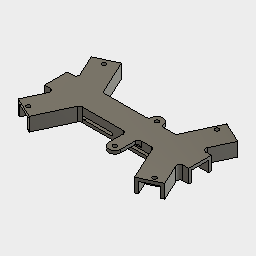
Central Frame V1.2 v4 (Autodesk Fusion 360 design; units mm, degrees)
Autodesk Fusion 360 part; units mm, degrees
sketch "Sketch1" plane through (0, 0, 0) normal (0, 1, 0) x (1, 0, 0)
  line L0 (13.8907, 50.6995) -> (18.8907, 50.6995) construction
  line L1 (13.8907, 50.6995) -> (21.3907, 50.6995) construction
  line L2 (20.688, 53.8691) -> (29.9066, 34.0997)
  line L3 (13.8907, 50.6995) -> (21.3907, 50.6995) construction
  line L4 (7.0934, 47.5298) -> (13.3559, 34.0997)
  line L5 (7.0934, 5.6696) -> (13.3559, 19.0997)
  line L6 (20.688, -0.6696) -> (29.9066, 19.0997)
  line L7 (7.0934, 47.5298) -> (4.9803, 52.0614)
  line L8 (7.0934, 47.5298) -> (12.0934, 47.5298) construction
  line L9 (4.9803, 52.0614) -> (18.5749, 58.4007)
  line L10 (20.688, 53.8691) -> (18.5749, 58.4007)
  line L11 (7.0934, 5.6696) -> (4.9803, 1.1381)
  line L12 (7.0934, 5.6696) -> (12.0934, 5.6696) construction
  line L13 (4.9803, 1.1381) -> (18.5749, -5.2012)
  line L14 (4.9803, 1.1381) -> (19.9803, 1.1381) construction
  line L15 (18.5749, -5.2012) -> (20.688, -0.6696)
  line L16 (13.3559, 34.0997) -> (13.3559, 19.0997)
  line L17 (96.6149, 2.5) -> (104.1149, 2.5) construction
  line L18 (85.1097, 49.1342) -> (78.099, 34.0997)
  line L19 (87.3176, -0.6696) -> (78.099, 19.0997)
  line L20 (94.6496, 34.0997) -> (94.6496, 19.0997)
  line L21 (100.9122, 5.6696) -> (94.6496, 19.0997)
  line L22 (100.9122, 47.5298) -> (94.6496, 34.0997)
  line L23 (103.0253, 52.0614) -> (89.4307, 58.4007)
  line L24 (100.9122, 47.5298) -> (103.0253, 52.0614)
  line L25 (87.3176, 53.8691) -> (89.4307, 58.4007)
  line L26 (100.9122, 5.6696) -> (103.0253, 1.1381)
  line L27 (103.0253, 1.1381) -> (89.4307, -5.2012)
  line L28 (89.4307, -5.2012) -> (87.3176, -0.6696)
  line L29 (29.9066, 34.0997) -> (60.3566, 34.0997)
  line L30 (68.3041, 34.0997) -> (78.099, 34.0997)
  arc A0 (68.3041, 35.3466) -> (60.3097, 35.3466) centre (64.3069, 35.4968) ccw
  line L31 (60.3097, 7.4466) -> (60.3097, 19.0997)
  line L32 (68.3069, 7.5968) -> (68.3069, 19.0997)
  arc A1 (60.3097, 7.747) -> (68.3069, 7.5968) centre (64.3069, 7.5968) ccw
  line L33 (29.9066, 19.0997) -> (60.3097, 19.0997)
  line L34 (68.3069, 19.0997) -> (78.099, 19.0997)
  line L35 (60.3097, 35.3466) -> (60.3566, 34.0997)
  line L36 (68.3041, 35.3466) -> (68.3041, 34.0989)
  line L37 (85.1097, 49.1342) -> (87.3176, 53.8691)
  dimension "d15" = 27.9
  dimension "d89" = 7.5
  dimension "d91" = 7.5
  dimension "d95" = 115
  dimension "d96" = 5
  dimension "d97" = 115
  dimension "d98" = 5
  dimension "d99" = 25
  dimension "d100" = 15
  dimension "d107" = 8
  dimension "d109" = 8
  dimension "d110" = 1.2478
  constraint horizontal L0
  constraint horizontal L1
  constraint horizontal L3
  constraint horizontal L8
  constraint perpendicular L2 L9
  constraint perpendicular L9 L10
  constraint horizontal L12
  constraint horizontal L14
  constraint perpendicular L13 L15
  constraint horizontal L29
  constraint horizontal L17
  constraint collinear L29 L30
  constraint coincident A1
  constraint perpendicular L31 L33
  constraint coincident origin L33
  constraint tangent L32 A1
  constraint perpendicular L32 L33
  constraint coincident L31
  constraint collinear L33 L34
  constraint tangent A0 L35
  constraint vertical L36
  constraint coincident L36
  constraint parallel L18 L37
  measures "d91" distance of origin
  measures "d95" angle of L7 L8
  measures "d97" angle of L11 L12
  measures "d98" distance of origin
  measures "d99" angle of L13 L14
  measures "d107" diameter of A0
  measures "d109" diameter of A1
  measures "d110" distance of origin
extrude "Extrude1" add sketch "Sketch1" along normal blind 2 contours L2 L4 L5 L6 L7 L9 L10 L11 L13 L15 L16 L18 L19 L20 L21 L22 L23 L24 L25 L26 L27 L28 L29 L30 A0 L31 L32 A1 L33 L34 L35 L36 L37
sketch "Sketch12" plane through (0, 2, 0) normal (0, 1, 0) x (-1, 0, 0)
  line L0 (-13.3559, -19.0997) -> (-4.9803, -1.1381)
  line L1 (-4.9803, -1.1381) -> (-18.5749, 5.2012)
  line L2 (-18.5749, 5.2012) -> (-29.9066, -19.0997)
  line L3 (-29.9066, -19.0997) -> (-60.3097, -19.0997)
  line L4 (-60.3097, -19.0997) -> (-60.3097, -7.4466)
  arc A0 (-60.3097, -7.4466) -> (-68.3069, -7.5968) centre (-64.3069, -7.5968) ccw
  line L5 (-68.3069, -7.5968) -> (-68.3069, -19.0997)
  line L6 (-68.3069, -19.0997) -> (-78.099, -19.0997)
  line L7 (-78.099, -19.0997) -> (-89.4307, 5.2012)
  line L8 (-89.4307, 5.2012) -> (-103.0253, -1.1381)
  line L9 (-103.0253, -1.1381) -> (-94.6496, -19.0997)
  line L10 (-94.6496, -19.0997) -> (-94.6496, -34.0997)
  line L11 (-94.6496, -34.0997) -> (-103.0253, -52.0614)
  line L12 (-103.0253, -52.0614) -> (-89.4307, -58.4007)
  line L13 (-89.4307, -58.4007) -> (-78.099, -34.0997)
  line L14 (-78.099, -34.0997) -> (-68.3041, -34.0997)
  line L15 (-68.3041, -34.0997) -> (-68.3041, -35.3466)
  arc A1 (-68.3041, -35.3466) -> (-60.3097, -35.3466) centre (-64.3069, -35.4968) ccw
  line L16 (-60.3097, -35.3466) -> (-60.3566, -34.0997)
  line L17 (-60.3566, -34.0997) -> (-29.9066, -34.0997)
  line L18 (-29.9066, -34.0997) -> (-18.5749, -58.4007)
  line L19 (-18.5749, -58.4007) -> (-4.9803, -52.0614)
  line L20 (-4.9803, -52.0614) -> (-13.3559, -34.0997)
  line L21 (-13.3559, -34.0997) -> (-13.3559, -19.0997)
  circle A2 centre (-13.0706, -1.5207) radius 1.3
  circle A3 centre (-13.8907, -50.6995) radius 1.3
  circle A4 centre (-64.3069, -7.5968) radius 1.3
  circle A5 centre (-64.3069, -35.4968) radius 1.3
  circle A6 centre (-88.7907, -50.6995) radius 1.3
  circle A7 centre (-95.7752, -2.3455) radius 1.3
  dimension "d193" = 2.6
  dimension "d194" = 2.6
  dimension "d195" = 2.6
  dimension "d196" = 2.6
  dimension "d197" = 2.6
  dimension "d198" = 2.6
  measures "d193" diameter of A2
  measures "d194" diameter of A3
  measures "d195" diameter of A4
  measures "d196" diameter of A5
  measures "d197" diameter of A6
  measures "d198" diameter of A7
extrude "Extrude10" cut sketch "Sketch12" against normal blind 2 contours A2 | A3 | A4 | A5 | A6 | A7
sketch "Sketch13" plane through (0, 0, 0) normal (0, -1, 0) x (1, 0, 0)
  line L0 (60.3566, -34.0997) -> (60.3097, -35.3466)
  arc A0 (60.3097, -35.3466) -> (68.3041, -35.3466) centre (64.3069, -35.4968) ccw
  line L1 (68.3041, -35.3466) -> (68.3041, -34.0997)
  line L2 (68.3041, -34.0997) -> (78.099, -34.0997)
  line L3 (78.099, -34.0997) -> (89.4307, -58.4007)
  line L4 (89.4307, -58.4007) -> (103.0253, -52.0614)
  line L5 (103.0253, -52.0614) -> (94.6496, -34.0997)
  line L6 (94.6496, -34.0997) -> (94.6496, -19.0997)
  line L7 (94.6496, -19.0997) -> (103.0253, -1.1381)
  line L8 (103.0253, -1.1381) -> (89.4307, 5.2012)
  line L9 (89.4307, 5.2012) -> (78.099, -19.0997)
  line L10 (78.099, -19.0997) -> (68.3069, -19.0997)
  line L11 (68.3069, -19.0997) -> (68.3069, -7.5968)
  arc A1 (68.3069, -7.5968) -> (60.3097, -7.4466) centre (64.3069, -7.5968) ccw
  line L12 (60.3097, -7.4466) -> (60.3097, -19.0997)
  line L13 (60.3097, -19.0997) -> (29.9066, -19.0997)
  line L14 (29.9066, -19.0997) -> (18.5749, 5.2012)
  line L15 (18.5749, 5.2012) -> (4.9803, -1.1381)
  line L16 (4.9803, -1.1381) -> (13.3559, -19.0997)
  line L17 (13.3559, -19.0997) -> (13.3559, -34.0997)
  line L18 (13.3559, -34.0997) -> (4.9803, -52.0614)
  line L19 (4.9803, -52.0614) -> (18.5749, -58.4007)
  line L20 (18.5749, -58.4007) -> (29.9066, -34.0997)
  line L21 (29.9066, -34.0997) -> (60.3566, -34.0997)
  line L22 (62.4331, -32.0997) -> (66.3041, -32.0997)
  line L23 (62.3097, -21.0997) -> (66.3069, -21.0997)
  line L24 (15.3559, -18.6563) -> (15.3559, -34.5431)
  line L25 (28.6325, -32.0997) -> (62.4331, -32.0997)
  line L26 (66.3041, -32.0997) -> (79.3731, -32.0997)
  line L27 (88.975, -52.691) -> (90.3981, -55.7428)
  line L28 (92.6496, -34.5431) -> (92.6496, -18.6563)
  line L29 (79.3731, -21.0997) -> (66.3069, -21.0997)
  line L30 (62.3097, -21.0997) -> (28.6325, -21.0997)
  line L31 (87.3836, -49.2782) -> (88.975, -52.691)
  line L32 (60.3566, -34.0997) -> (68.3041, -34.0997)
  line L33 (60.3097, -19.0997) -> (68.3069, -19.0997)
  line L34 (7.6381, -51.094) -> (6.7929, -52.9066)
  line L35 (17.6075, -55.7428) -> (16.7623, -57.5554)
  line L36 (17.6075, -55.7428) -> (19.6075, -55.7428) construction
  line L37 (7.6381, -2.1055) -> (6.7929, -0.2929)
  line L38 (17.6075, 2.5433) -> (16.7623, 4.3559)
  line L39 (17.6075, 2.5433) -> (19.6075, 2.5433) construction
  line L40 (90.3981, 2.5433) -> (91.2433, 4.3559)
  line L41 (90.3981, 2.5433) -> (92.3981, 2.5433) construction
  line L42 (100.3674, -2.1055) -> (101.2127, -0.2929)
  line L43 (100.3674, -2.1055) -> (102.3674, -2.1055) construction
  line L44 (90.3981, -55.7428) -> (91.2433, -57.5554)
  line L45 (90.3981, -55.7428) -> (92.3981, -55.7428) construction
  line L46 (100.3674, -51.094) -> (101.2127, -52.9066)
  line L47 (6.7929, -0.2929) -> (11.0191, -9.3559)
  line L48 (6.7929, -0.2929) -> (16.7929, -0.2929) construction
  line L49 (11.0191, -9.3559) -> (20.9885, -4.7071)
  line L50 (6.7929, -52.9066) -> (11.0191, -43.8435)
  line L51 (6.7929, -52.9066) -> (16.7929, -52.9066) construction
  line L52 (11.0191, -43.8435) -> (20.9885, -48.4923)
  line L53 (91.2433, 4.3559) -> (87.0171, -4.7071)
  line L54 (87.0171, -4.7071) -> (96.9865, -9.3559)
  line L55 (101.2127, -52.9066) -> (96.9865, -43.8435)
  line L56 (101.2127, -52.9066) -> (111.2127, -52.9066) construction
  line L57 (96.9865, -43.8435) -> (87.0171, -48.4923)
  line L58 (11.497, -42.8186) -> (21.4664, -47.4674)
  line L59 (11.497, -10.3809) -> (21.4664, -5.7321)
  line L60 (86.5392, -5.7321) -> (96.5085, -10.3809)
  line L61 (96.5085, -42.8186) -> (86.5392, -47.4674)
  line L62 (17.6075, -55.7428) -> (20.9885, -48.4923)
  line L63 (21.4664, -47.4674) -> (28.6325, -32.0997)
  line L64 (15.3559, -34.5431) -> (11.497, -42.8186)
  line L65 (11.0191, -43.8435) -> (7.6381, -51.094)
  line L66 (7.6381, -2.1055) -> (11.0191, -9.3559)
  line L67 (11.497, -10.3809) -> (15.3559, -18.6563)
  line L68 (28.6325, -21.0997) -> (21.4664, -5.7321)
  line L69 (20.9885, -4.7071) -> (17.6075, 2.5433)
  line L70 (90.3981, 2.5433) -> (87.0171, -4.7071)
  line L71 (86.5392, -5.7321) -> (79.3731, -21.0997)
  line L72 (92.6496, -18.6563) -> (96.5085, -10.3809)
  line L73 (96.9865, -9.3559) -> (100.3674, -2.1055)
  line L74 (100.3674, -51.094) -> (96.9865, -43.8435)
  line L75 (96.5085, -42.8186) -> (92.6496, -34.5431)
  line L76 (79.3731, -32.0997) -> (86.5392, -47.4674)
  line L77 (87.0171, -48.4923) -> (87.3836, -49.2782)
  circle A2 centre (88.7907, -50.6995) radius 1.3
  circle A3 centre (13.0706, -1.5207) radius 1.3
  circle A4 centre (64.3069, -35.4968) radius 1.3
  circle A5 centre (95.7752, -2.3455) radius 1.3
  circle A6 centre (64.3069, -7.5968) radius 1.3
  circle A7 centre (13.8907, -50.6995) radius 1.3
  dimension "d131" = 115
  dimension "d132" = 2
  dimension "d133" = 115
  dimension "d134" = 2
  dimension "d135" = 115
  dimension "d136" = 2
  dimension "d137" = 65
  dimension "d138" = 2
  dimension "d139" = 65
  dimension "d140" = 2
  dimension "d141" = 65
  dimension "d142" = 2
  dimension "d143" = 65
  dimension "d144" = 10
  dimension "d145" = 65
  dimension "d146" = 10
  dimension "d147" = 10
  dimension "d148" = 115
  dimension "d149" = 10
  constraint parallel L16 L66
  constraint parallel L17 L24
  constraint parallel L18 L64
  constraint parallel L20 L62
  constraint parallel L21 L25
  constraint parallel L2 L26
  constraint parallel L3 L27
  constraint parallel L5 L74
  constraint parallel L6 L28
  constraint parallel L7 L72
  constraint parallel L9 L70
  constraint parallel L10 L29
  constraint parallel L13 L30
  constraint parallel L14 L68
  constraint parallel L27 L31
  constraint coincident L19 origin
  constraint horizontal L36
  constraint horizontal L39
  constraint horizontal L41
  constraint horizontal L43
  constraint horizontal L45
  constraint coincident L4 origin
  constraint horizontal L48
  constraint coincident origin L68
  constraint perpendicular L49 L68
  constraint horizontal L51
  constraint perpendicular L52 L62
  constraint coincident L72
  constraint perpendicular L54 L72
  constraint horizontal L56
  constraint coincident origin L76
  constraint perpendicular L57 L76
  constraint coincident origin L62
  constraint perpendicular L58 L62
  constraint perpendicular L59 L66
  constraint coincident L70
  constraint perpendicular L60 L72
  constraint perpendicular L61 L76
  constraint collinear L62 L63
  constraint collinear L64 L65
  constraint collinear L66 L67
  constraint coincident L66
  constraint collinear L68 L69
  constraint collinear L70 L71
  constraint collinear L72 L73
  constraint collinear L74 L75
  constraint coincident L74
  constraint collinear L76 L77
  measures "d131" angle of L35 L36
  measures "d133" angle of L36 L37
  measures "d135" angle of L38 L39
  measures "d137" angle of L40 L41
  measures "d139" angle of L42 L43
  measures "d140" distance of origin
  measures "d141" angle of L44 L45
  measures "d143" angle of L47 L48
  measures "d145" angle of L50 L51
  measures "d147" distance of origin
  measures "d148" angle of L55 L56
extrude "Extrude11" add sketch "Sketch13" along normal blind 7 contours L2 L3 L4 L5 L6 L7 L8 L9 L10 L13 L14 L15 L16 L17 L18 L19 L20 L21 L27 L31 L32 L33 L34 L35 L37 L38 L40 L42 L44 L46 L47 L49 L50 L52 L53 L54 L55 L57 L62 L65 L66 L69 L70 L73 L74 L77 A2 | L31 A2 picked at (87.9233, -50.8802)
sketch "Sketch18" plane through (0, 0, -19.0997) normal (0, 0, 1) x (1, 0, 0)
  line L0 (60.3097, 2) -> (29.9066, 2)
  line L1 (68.3069, 0) -> (60.3097, 0)
  line L2 (29.9066, -7) -> (78.099, -7)
  line L3 (51.5025, -5) -> (31.5025, -5)
  line L4 (31.5025, -5) -> (31.5025, -3)
  line L5 (31.5025, -3) -> (51.5025, -3)
  line L6 (51.5025, -3) -> (51.5025, -5)
  line L7 (56.5025, -5) -> (76.5025, -5)
  line L8 (76.5025, -5) -> (76.5025, -3)
  line L9 (76.5025, -3) -> (56.5025, -3)
  line L10 (56.5025, -3) -> (56.5025, -5)
  line L11 (60.3097, 0) -> (60.3097, 2)
  line L12 (29.9066, 2) -> (29.9066, -7)
  line L13 (78.099, -7) -> (78.099, 2)
  line L14 (78.099, 2) -> (68.3069, 2)
  line L15 (68.3069, 2) -> (68.3069, 0)
  dimension "d180" = 20
  dimension "d181" = 2
  dimension "d182" = 2
  dimension "d183" = 20
  constraint horizontal L3
  constraint vertical L4
  constraint horizontal L5
  constraint vertical L6
  constraint horizontal L7
  constraint vertical L8
  constraint horizontal L9
  constraint vertical L10
  measures "d181" distance of origin
  measures "d182" distance of origin
extrude "Extrude13" cut sketch "Sketch18" against normal blind 15 contours L3 L4 L5 L6 | L7 L8 L9 L10
fillet "Fillet10" radius 1 16 edges at (51.5025, -3, -20.0997) (31.5025, -5, -20.0997) (51.5025, -5, -20.0997) (56.5025, -5, -20.0997) (56.5025, -3, -20.0997) (76.5025, -3, -20.0997) (76.5025, -5, -20.0997) (56.5025, -3, -33.0997) (56.5025, -5, -33.0997) (51.5025, -3, -33.0997) (51.5025, -5, -33.0997) (31.5025, -3, -33.0997) (31.5025, -5, -33.0997) (76.5025, -3, -33.0997) (76.5025, -5, -33.0997) (31.5025, -3, -20.0997)
sketch "Sketch19" plane through (0, 2, 0) normal (0, 1, 0) x (-1, 0, 0)
  line L0 (-78.099, -34.0997) -> (-68.3041, -34.0997)
  line L1 (-29.9066, -34.0997) -> (-18.5749, -58.4007)
  line L2 (-18.5749, -58.4007) -> (-4.9803, -52.0614)
  line L3 (-4.9803, -52.0614) -> (-13.3559, -34.0997)
  line L4 (-13.3559, -34.0997) -> (-13.3559, -19.0997)
  line L5 (-13.3559, -19.0997) -> (-4.9803, -1.1381)
  line L6 (-4.9803, -1.1381) -> (-18.5749, 5.2012)
  line L7 (-18.5749, 5.2012) -> (-29.9066, -19.0997)
  line L8 (-29.9066, -19.0997) -> (-60.3097, -19.0997)
  line L9 (-60.3097, -19.0997) -> (-60.3097, -7.4466)
  arc A0 (-60.3097, -7.4466) -> (-68.3069, -7.5968) centre (-64.3069, -7.5968) ccw
  line L10 (-68.3069, -7.5968) -> (-68.3069, -19.0997)
  line L11 (-78.099, -19.0997) -> (-89.4307, 5.2012)
  line L12 (-89.4307, 5.2012) -> (-103.0253, -1.1381)
  line L13 (-103.0253, -1.1381) -> (-94.6496, -19.0997)
  line L14 (-94.6496, -19.0997) -> (-94.6496, -34.0997)
  line L15 (-94.6496, -34.0997) -> (-103.0253, -52.0614)
  line L16 (-103.0253, -52.0614) -> (-89.4307, -58.4007)
  line L17 (-89.4307, -58.4007) -> (-78.099, -34.0997)
  arc A1 (-68.3041, -35.3466) -> (-60.3097, -35.3466) centre (-64.3069, -35.4968) ccw
  line L18 (-4.9803, -1.1381) -> (-18.5749, 5.2012)
  line L19 (-18.5749, 5.2012) -> (-19.2088, 3.8417)
  line L20 (-19.2088, 3.8417) -> (-5.6142, -2.4976)
  line L21 (-5.6142, -2.4976) -> (-4.9803, -1.1381)
  line L22 (-4.9803, -52.0614) -> (-18.5749, -58.4007)
  line L23 (-18.5749, -58.4007) -> (-19.2088, -57.0412)
  line L24 (-19.2088, -57.0412) -> (-5.6142, -50.7019)
  line L25 (-5.6142, -50.7019) -> (-4.9803, -52.0614)
  line L26 (-89.4307, -58.4007) -> (-103.0253, -52.0614)
  line L27 (-103.0253, -52.0614) -> (-102.3914, -50.7019)
  line L28 (-102.3914, -50.7019) -> (-88.7968, -57.0412)
  line L29 (-88.7968, -57.0412) -> (-89.4307, -58.4007)
  line L30 (-89.4307, 5.2012) -> (-103.0253, -1.1381)
  line L31 (-103.0253, -1.1381) -> (-102.3914, -2.4976)
  line L32 (-102.3914, -2.4976) -> (-88.7968, 3.8417)
  line L33 (-88.7968, 3.8417) -> (-89.4307, 5.2012)
  circle A2 centre (-13.8907, -50.6995) radius 1.3
  circle A3 centre (-64.3069, -7.5968) radius 1.3
  circle A4 centre (-95.7752, -2.3455) radius 1.3
  circle A5 centre (-13.0706, -1.5207) radius 1.3
  circle A6 centre (-88.7907, -50.6995) radius 1.3
  circle A7 centre (-64.3069, -35.4968) radius 1.3
  line L34 (-68.3069, -19.0997) -> (-78.099, -19.0997)
  line L35 (-68.3041, -34.0997) -> (-68.3041, -35.3466)
  line L36 (-60.3097, -35.3466) -> (-60.3566, -34.0997)
  line L37 (-60.3566, -34.0997) -> (-29.9066, -34.0997)
  dimension "d187" = 1.5
  dimension "d188" = 1.5
  dimension "d189" = 1.5
  dimension "d190" = 1.5
  constraint perpendicular L18 L19
  constraint parallel L18 L20
  constraint parallel L19 L21
  constraint perpendicular L7 L18
  constraint perpendicular L22 L23
  constraint parallel L22 L24
  constraint parallel L23 L25
  constraint perpendicular L1 L22
  constraint perpendicular L26 L27
  constraint parallel L26 L28
  constraint parallel L27 L29
  constraint perpendicular L15 L26
  constraint perpendicular L30 L31
  constraint parallel L30 L32
  constraint parallel L31 L33
  constraint perpendicular L13 L30
  measures "d187" distance of origin
  measures "d190" distance of origin
extrude "Extrude14" cut sketch "Sketch19" against normal blind 9 contours L15 L16 L17 L26 L27 L28 L29 | L11 L12 L13 L30 L31 L32 L33 | L1 L2 L3 L22 L23 L24 L25 | L5 L6 L7 L18 L19 L20 L21
sketch "Sketch23" plane through (94.6496, 0, 0) normal (1, 0, 0) x (0, 0, -1)
  line L0 (19.0997, -7) -> (34.0997, -7)
  line L1 (34.0997, 2) -> (19.0997, 2)
  line L2 (34.0997, -7) -> (34.0997, 2)
  line L3 (19.0997, 2) -> (19.0997, -7)
  line L4 (19.0997, 2) -> (34.0997, 2)
  line L5 (34.0997, 2) -> (34.0997, -7)
  line L6 (34.0997, -7) -> (19.0997, -7)
  line L7 (19.0997, -7) -> (19.0997, 2)
  line L8 (32.0997, 0) -> (32.0997, -5)
  line L9 (21.0997, -5) -> (21.0997, 0)
  line L10 (21.0997, 0) -> (32.0997, 0)
  line L11 (21.0997, -5) -> (21.0997, -7)
  line L12 (32.0997, -5) -> (32.0997, -7)
  constraint horizontal L4
  constraint vertical L5
  constraint horizontal L6
  constraint vertical L7
  constraint parallel L5 L8
  constraint parallel L7 L9
  constraint parallel L4 L10
  constraint perpendicular L6 L11
  constraint perpendicular L6 L12
extrude "Extrude15" add sketch "Sketch23" along normal blind 7 contours L0 L1 L2 L3 L4 L5 L6 L7 L8 L9 L10 L11 L12
sketch "Sketch24" plane through (13.3559, 0, 0) normal (-1, 0, 0) x (0, 0, 1)
  line L0 (-19.0997, -7) -> (-19.0997, 2)
  line L1 (-19.0997, 2) -> (-34.0997, 2)
  line L2 (-34.0997, 2) -> (-34.0997, -7)
  line L3 (-34.0997, -7) -> (-19.0997, -7)
  line L4 (-34.0997, 2) -> (-19.0997, 2)
  line L5 (-19.0997, 2) -> (-19.0997, -7)
  line L6 (-19.0997, -7) -> (-34.0997, -7)
  line L7 (-34.0997, -7) -> (-34.0997, 2)
  line L8 (-32.0997, -5) -> (-32.0997, 0)
  line L9 (-32.0997, 0) -> (-21.0997, 0)
  line L10 (-21.0997, 0) -> (-21.0997, -5)
  line L11 (-32.0997, -5) -> (-32.0997, -7)
  line L12 (-21.0997, -5) -> (-21.0997, -7)
  constraint horizontal L4
  constraint vertical L5
  constraint horizontal L6
  constraint vertical L7
  constraint parallel L7 L8
  constraint parallel L4 L9
  constraint parallel L5 L10
  constraint perpendicular L6 L11
  constraint perpendicular L6 L12
extrude "Extrude16" add sketch "Sketch24" along normal blind 7 contours L0 L1 L2 L3 L4 L5 L6 L7 L8 L9 L10 L11 L12
fillet "Fillet11" radius 2 4 edges at (13.3559, -2.5, -19.0997) (13.3559, -2.5, -34.0997) (94.6496, -2.5, -34.0997) (94.6496, -2.5, -19.0997)
fillet "Fillet13" radius 2 9 edges at (64.3083, 0, -19.0997) (68.3069, 1, -19.0997) (60.3097, 1, -19.0997) (68.3041, 1, -34.0997) (60.3566, 1, -34.0997) (29.9066, -2.5, -19.0997) (78.099, -2.5, -19.0997) (78.099, -2.5, -34.0997) (29.9066, -2.5, -34.0997)
